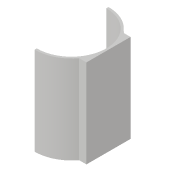
# Autodesk Inventor part: BlockSlideTestTube
Saved by Autodesk Inventor 2018 (Build 220112000, 112)
## iProperties
Created: 2018-12-13
Part Number: BlockSlideTestTube
Material: Generic
Document SubType Name: Modeling
Designer: ball
Density: 1 g/cm^3
Appearance: Default
Author: ball
Autodesk Inventor part; units mm, degrees
ref_plane "YZ Plane" through (0, 0, 0) normal (1, 0, 0) x (0, 1, 0)
ref_plane "XZ Plane" through (0, 0, 0) normal (0, 1, 0) x (-1, 0, 0)
ref_plane "XY Plane" through (0, 0, 0) normal (0, 0, 1) x (1, 0, 0)
sketch "Sketch1" plane through (0, 0, 0) normal (0, 1, 0) x (-1, 0, 0)
  arc A0 (0, 42.545) -> (0, -42.545) centre (0, 0) ccw
  arc A1 (0, 40.005) -> (0, -40.005) centre (0, 0) ccw
  line L0 (0, 42.545) -> (0, 40.005)
  line L1 (0, -40.005) -> (0, -42.545)
  line L2 (-40.005, 0) -> (-42.545, 0)
  line L3 (-42.545, 0) -> (-42.545, -25.4)
  line L4 (-42.545, -25.4) -> (-34.1309, -25.4)
  line L5 (-40.005, 0) -> (-42.545, 0)
  line L6 (-42.545, 0) -> (-42.545, 25.4)
  line L7 (-42.545, 25.4) -> (-34.1309, 25.4)
  dimension "d0" = 85.09
  dimension "d1" = 80.01
  dimension "d2" = 25.4
  dimension "d3" = 25.4
  constraints: 16 end point, 9 point on circle, 2 centre point, 2 coincident, 2 horizontal, 2 parallel, 2 perpendicular, 1 collinear, 1 point on line
  measures "d0" diameter of A0
  measures "d1" diameter of A1
  measures "d2" distance of L3.end L2.end
  measures "d3" distance of L5.end L6.end
extrude "Extrusion1" add sketch "Sketch1" along normal blind 101.6
body "Solid1"
